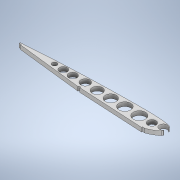
# Autodesk Inventor part: airfoil
Saved by Autodesk Inventor 2022 (Build 260153000, 153)
## iProperties
Created: 2021-03-06
Part Number: airfoil
Material: Generic
Document SubType Name: Modeling
Designer: Ferdinand Hubbard
Density: 1 g/cm^3
Appearance: Default
Author: Ferdinand Hubbard
Autodesk Inventor part; units mm, degrees
ref_plane "YZ Plane" through (0, 0, 0) normal (1, 0, 0) x (0, 1, 0)
ref_plane "XZ Plane" through (0, 0, 0) normal (0, 1, 0) x (-1, 0, 0)
ref_plane "XY Plane" through (0, 0, 0) normal (0, 0, 1) x (1, 0, 0)
sketch "Sketch1" plane through (0, 0, 0) normal (0, 1, 0) x (-1, 0, 0)
  circle A0 centre (139.2211, 7.3389) radius 13.5
  circle A1 centre (104.5253, 7.6129) radius 14.5
  circle A2 centre (172.6846, 7.1168) radius 12.5
  circle A3 centre (258.2615, 4.8535) radius 8
  circle A4 centre (67.3128, 9.1933) radius 15
  spline S0 degree 4 poles (39.9436, 31.3088) (37.7662, 30.6563) (33.258, 29.1761) (27.1595, 26.7117) (19.6138, 22.8804) (11.2549, 17.3272) (6.0635, 12.605) (2.8423, 8.0332) (1.9781, 6.5051) knots 0.209844 0.209844 0.209844 0.209844 0.209844 0.338648 0.479254 0.612645 0.738339 1 1 1 1 1
  circle A5 centre (36.5825, 9.1521) radius 10
  circle A6 centre (281.2667, 3.3987) radius 6
  line L0 (229.1022, 19.6309) -> (363.9286, 4.3933)
  circle A7 centre (370.8333, 3.6129) radius 4 construction
  circle A8 centre (234.2487, 5.7058) radius 10
  spline S1 degree 4 poles (6.5182, -5.2336) (7.1494, -5.5885) (14.4657, -7.5137) (22.7137, -8.712) (35.9318, -9.9587) (48.9047, -10.4891) (62.2875, -10.9022) (78.073, -11.0572) (94.7047, -11.0677) (112.5814, -10.9206) (131.2146, -10.6478) (157.2989, -10.1249) (178.3611, -9.5706) (196.5094, -9.0102) (204.4618, -8.7595) knots 0 0 0 0 0 0.111054 0.172284 0.238398 0.309093 0.3838 0.461605 0.542502 0.625628 0.710437 0.796395 1 1 1 1 1
  arc A9 (204.8781, 22.3686) -> (204.3228, 22.4313) centre (203.7026, 14.4554) ccw
  line L1 (204.4618, -8.7595) -> (204.4618, -8.7595) construction
  arc A10 (204.4618, -8.7595) -> (204.4618, -8.7595) centre (-110.5763, 9986.2768) ccw construction
  line L2 (204.3228, 22.4313) -> (205.1008, 22.3434)
  arc A11 (366.8584, 4.0604) -> (366.7756, 4.0715) centre (366.551, 2.0842) ccw
  line L3 (205.1008, 22.3434) -> (229.1022, 19.6309)
  line L4 (204.4618, -8.7595) -> (226.4407, -8.0668)
  circle A12 centre (13.7691, 4.0715) radius 9.5
  circle A13 centre (13.7691, 4.0715) radius 8
  line L5 (6.5181, 10.2093) -> (6.4686, 10.2474)
  line L6 (6.5181, -2.0663) -> (6.4883, -2.0926)
  line L7 (6.3756, -3.4733) -> (8.2772, -5.8071)
  line L8 (6.2475, 11.5973) -> (7.6237, 13.6489)
  line L9 (7.6236, 9.1933) -> (7.4154, 9.3611)
  line L10 (7.111, 10.5032) -> (8.7725, 14.7639)
  line L11 (7.7077, -1.1495) -> (7.655, -1.1924)
  line L12 (7.6239, -2.4061) -> (12.536, -6.8462)
  arc A14 (6.4883, -2.0926) -> (6.3756, -3.4733) centre (7.1509, -2.8416) ccw
  arc A15 (7.655, -1.1924) -> (7.6239, -2.4061) centre (8.1603, -1.8126) ccw
  arc A16 (7.111, 10.5032) -> (7.4154, 9.3611) centre (8.0427, 10.1399) ccw
  arc A17 (6.2475, 11.5973) -> (6.4686, 10.2474) centre (7.078, 11.0402) ccw
  circle A18 centre (204.3228, 4.8389) radius 11
  circle A19 centre (258.2615, 4.8535) radius 9.5
  line L13 (199.7021, 25.262) -> (204.7021, 25.262)
  line L14 (204.7021, 25.262) -> (204.7021, 20.262)
  line L15 (204.7021, 20.262) -> (199.7021, 20.262)
  line L16 (199.7021, 20.262) -> (199.7021, 25.262)
  line L17 (34.9436, 34.0508) -> (39.9436, 34.0508)
  line L18 (39.9436, 34.0508) -> (39.9436, 29.0508)
  line L19 (39.9436, 29.0508) -> (34.9436, 29.0508)
  line L20 (34.9436, 29.0508) -> (34.9436, 34.0508)
  line L21 (46.0738, 33.1455) -> (33.8135, 29.472) construction
  arc A20 (44.8753, 32.6689) -> (35.0766, 29.7329) centre (73.296, -80.0039) ccw construction
  line L22 (39.9436, 31.3088) -> (204.3228, 22.4313)
  line L23 (363.9286, 7.3389) -> (368.9286, 7.3389)
  line L24 (368.9286, 7.3389) -> (368.9286, 2.3389)
  line L25 (368.9286, 2.3389) -> (363.9286, 2.3389)
  line L26 (363.9286, 2.3389) -> (363.9286, 7.3389)
  line L27 (368.9286, 2.3389) -> (368.9286, 1.9316)
  arc A21 (366.9727, -0.0679) -> (368.9286, 1.9316) centre (366.9286, 1.9316) ccw
  spline S2 degree 4 poles (226.4407, -8.0668) (226.7168, -7.9106) (246.397, -7.271) (261.9174, -6.5757) (283.9748, -5.5203) (299.9172, -4.5963) (314.7263, -3.6143) (328.2274, -2.6448) (339.6733, -1.7771) (350.204, -1.0417) (357.3568, -0.5279) (364.7416, -0.1778) (365.8834, -0.1194) (366.8566, -0.0835) knots 0 0 0 0 0 0.209603 0.316305 0.419804 0.519462 0.614592 0.704374 0.787764 0.863385 0.925581 1 1 1 1 1
  spline S3 degree 4 poles (369.983, -0.0016) (369.9988, -0.0007) (370.0055, 0.0002) (370.0019, 0.001) (369.9872, 0.0018) knots 0 0 0 0 0 1 1 1 1 1
  line L28 (369.9445, -0.0037) -> (370.0215, 0.0006) construction
  arc A22 (369.9522, -0.0026) -> (370.0137, 0.0008) centre (369.9433, 0.7095) ccw construction
  line L29 (366.9727, -0.0679) -> (366.8566, -0.0835)
  line L30 (352.3876, -0.6183) -> (381.3257, 0.4513) construction
  arc A23 (378.4115, -0.1225) -> (355.3362, -0.9754) centre (372.1508, -143.3164) ccw construction
  point P0 (0, 0)
  point P1 (19.2974, 22.4624)
  point P2 (12.8156, 18.139)
  point P3 (3.7499, 9.1521)
  point P4 (1.2115, 4.8535)
  point P5 (0.0668, 1.0195)
  point P6 (0.0003, -0.0638)
  point P7 (0.0755, -0.9849)
  point P8 (0.2106, -1.5356)
  point P9 (0.4302, -2.0122)
  point P10 (0.7739, -2.4345)
  point P11 (1.2488, -2.8423)
  point P12 (2.1566, -3.4383)
  point P13 (3.2773, -4.0196)
  point P14 (15.3669, -7.4261)
  point P15 (24.3167, -8.7706)
  point P16 (35.0526, -9.7678)
  point P17 (47.9909, -10.4262)
  point P18 (61.6814, -10.8267)
  point P19 (77.2847, -11.0213)
  point P20 (94.162, -11.0379)
  point P21 (112.1091, -10.9014)
  point P22 (130.911, -10.6315)
  point P23 (150.3435, -10.2474)
  point P24 (170.176, -9.7646)
  point P25 (190.1737, -9.1986)
  point P26 (210.9592, -8.8383)
  point P27 (248.7963, -7.1166)
  point P28 (267.1071, -6.3194)
  point P29 (284.4371, -5.4606)
  point P30 (300.619, -4.5258)
  point P31 (315.5184, -3.5432)
  point P32 (328.988, -2.5786)
  point P33 (340.8625, -1.7041)
  point P34 (350.9622, -0.9861)
  point P35 (359.0984, -0.4682)
  point P36 (365.0855, -0.1602)
  point P37 (368.7597, -0.0285)
  point P38 (112.1091, -11.9485)
  point P39 (1.9781, 6.5051)
  point P40 (204.4618, -8.7595)
  point P41 (5.7252, 10.8187)
  point P42 (5.7691, -2.7289)
  point P43 (6.8449, 9.8206)
  point P44 (6.9324, -1.7811)
  point P45 (46.0163, 32.9548)
  point P46 (369.983, -0.0016)
  point P47 (204.7021, 22.3885)
  point P48 (199.7021, 22.6809)
  point P49 (34.9436, 29.6802)
  point P50 (204.4618, -8.7595)
  dimension "d69" = 8
  dimension "d50" = 368.7594
  dimension "d57" = 16
  dimension "d70" = 20
  dimension "d80" = 19
  dimension "d81" = 16
  dimension "d82" = 1
  dimension "d83" = 1
  dimension "d84" = 1
  dimension "d85" = 1
  dimension "d86" = 1
  dimension "d87" = 0.8
  dimension "d88" = 1
  dimension "d90" = 19
  dimension "d94" = 5
  dimension "d95" = 5
  dimension "d101" = 5
  dimension "d102" = 5
  dimension "d105" = 5
  dimension "d106" = 5
  dimension "d108" = 2
  dimension "d109" = 22
  dimension "d110" = 30
  dimension "d111" = 29
  dimension "d112" = 27
  dimension "d113" = 25
  constraints: 62 end point, 23 centre point, 22 point on circle, 12 point on line, 10 tangent, 8 midpoint, 6 parallel, 3 coincident, 3 horizontal, 3 perpendicular, 1 collinear, 1 equal radius, 52 other
  measures "d50" distance of point (368.76, -0.028) point (0, -0.064)
  measures "d57" diameter of A3
  measures "d70" diameter of A8
  measures "d80" diameter of A12
  measures "d81" diameter of A13
  measures "d82" distance of L5.start point (5.725, 10.819)
  measures "d83" distance of L6.start point (5.769, -2.729)
  measures "d84" distance of L9.start point (6.845, 9.821)
  measures "d85" distance of L11.start point (6.932, -1.781)
  measures "d86" radius of A14
  measures "d87" radius of A15
  measures "d88" radius of A16
  measures "d90" diameter of A19
  measures "d94" distance of L14.end L15.end
  measures "d95" distance of L13.end L14.end
  measures "d101" distance of L18.end L19.end
  measures "d102" distance of L17.end L18.end
  measures "d105" distance of L24.end L25.end
  measures "d106" distance of L23.end L24.end
  measures "d108" radius of A21
  measures "d109" diameter of A18
  measures "d110" diameter of A4
  measures "d111" diameter of A1
  measures "d112" diameter of A0
  measures "d113" diameter of A2
extrude "Extrusion5" add sketch "Sketch1" along normal blind 10 contours L10 A12 L5 A17 L8 S0 | S0 L20 L19 L18 L22 L16 L15 L14 A9 L2 L3 L0 L26 L25 L27 A21 L29 S2 L4 S1 L12 A12 L10 | L12 S1 L7 A14 L6 A12
body "Solid5"
